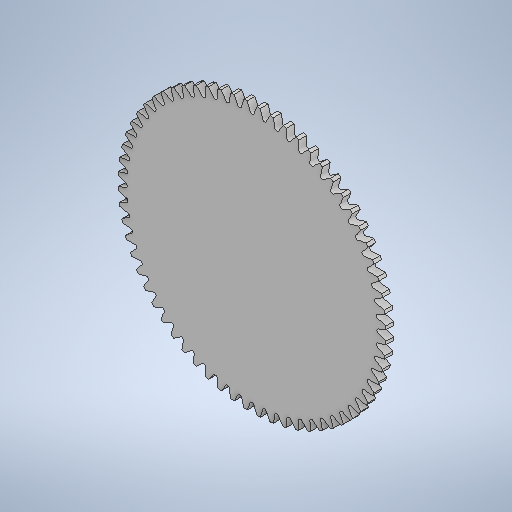
# Autodesk Inventor part: big gear
Saved by Autodesk Inventor 2025 (Build 290162010, 162A)
## iProperties
Created: 2025-08-27
Part Number: big gear
Material: Generic
Document SubType Name: Modeling
Designer: pokla
Density: 1 g/cm^3
Appearance: Default
Author: pokla
Autodesk Inventor part; units mm, degrees
ref_plane "YZ Plane" through (0, 0, 0) normal (1, 0, 0) x (0, 1, 0)
ref_plane "XZ Plane" through (0, 0, 0) normal (0, 1, 0) x (-1, 0, 0)
ref_plane "XY Plane" through (0, 0, 0) normal (0, 0, 1) x (1, 0, 0)
sketch "Sketch1" plane through (0, 0, 0) normal (0, 0, 1) x (1, 0, 0)
  spline S0 degree 3 poles (-15.3136, 412.2157) (-14.7005, 410.9627) (-13.4744, 408.4567) (-11.7613, 404.6382) (-10.1461, 400.7772) (-8.6557, 396.867) (-7.2691, 392.9165) (-6.406, 389.9001) (-5.7884, 387.899) (-5.3377, 386.951) (-4.8395, 386.2299) (-4.359, 385.7235) (-3.8332, 385.2647) (-3.236, 384.8928) (-2.5894, 384.6288) (-2.0848, 384.4891) (-1.5698, 384.3899) (-0.8714, 384.3654) (0, 384.3814) (0.8714, 384.3654) (1.5698, 384.3899) (2.0848, 384.4891) (2.5894, 384.6288) (3.236, 384.8928) (3.8332, 385.2647) (4.359, 385.7235) (4.8395, 386.2299) (5.3377, 386.951) (5.7884, 387.899) (6.406, 389.9001) (7.2691, 392.9165) (8.6557, 396.867) (10.1461, 400.7772) (11.7613, 404.6382) (13.4744, 408.4567) (14.7005, 410.9627) (15.3136, 412.2157) knots 0 0 0 0 0.418453 0.836906 1.255357 1.673806 2.09225 2.510695 2.615288 2.719831 2.824322 2.876636 2.92893 3.033403 3.085707 3.138007 3.190298 3.242598 3.347213 3.451829 3.504129 3.55642 3.60872 3.661023 3.765497 3.817791 3.870105 3.974596 4.079139 4.183732 4.602176 5.020621 5.43907 5.857521 6.275974 6.694427 6.694427 6.694427 6.694427
  circle A0 centre (0, 0) radius 384.375 construction
  circle A1 centre (0, 0) radius 375.877 construction
  circle A2 centre (0, 0) radius 400 construction
  circle A3 centre (0, 0) radius 412.5
  point P0 (-13.4954, 408.4468)
  point P1 (-11.7776, 404.6311)
  point P2 (-10.1669, 400.769)
  point P3 (-8.673, 396.8603)
  point P4 (-7.3084, 392.9046)
  point P5 (-6.0957, 388.8997)
  point P6 (-5.7647, 387.9075)
  point P7 (-5.3131, 386.9647)
  point P8 (-4.7127, 386.1094)
  point P9 (-4.3533, 385.7294)
  point P10 (-3.9585, 385.3864)
  point P11 (-3.0706, 384.8359)
  point P12 (-2.5862, 384.6385)
  point P13 (-2.083, 384.4958)
  point P14 (-1.5684, 384.4034)
  point P15 (-1.0462, 384.3746)
  point P16 (0, 384.375)
  point P17 (1.0462, 384.3746)
  point P18 (1.5684, 384.4034)
  point P19 (2.083, 384.4958)
  point P20 (2.5862, 384.6385)
  point P21 (3.0706, 384.8359)
  point P22 (3.9585, 385.3864)
  point P23 (4.3533, 385.7294)
  point P24 (4.7127, 386.1094)
  point P25 (5.3131, 386.9647)
  point P26 (5.7647, 387.9075)
  point P27 (6.0957, 388.8997)
  point P28 (7.3084, 392.9046)
  point P29 (8.673, 396.8603)
  point P30 (10.1669, 400.769)
  point P31 (11.7776, 404.6311)
  point P32 (13.4954, 408.4468)
  constraints: 4 centre point, 2 point on circle, 75 other
extrude "Extrusion1" add sketch "Sketch1" against normal blind 24
extrude "Extrusion2" cut sketch "Sketch1" against normal through all contours A3 S0 picked at (-1.5801, 403.5429)
pattern_circular "Circular Pattern1" count 64 over 360 about axis through (0, 0, -10) along (0, 0, 1) of "Extrusion2"
equation "\"Module\" = 12.5"
equation "\"PressureAngle\" = 20deg"
equation "\"UnitProfileClearance\" = 0.25"
equation "\"UnitRoundRadius\" = 0.35"
equation "\"HeadDiameter\" = 825"
equation "\"RootDiameter\" = 768.75"
equation "\"BaseDiameter\" = 751.7541"
equation "\"HelixAngle\" = 0"
equation "\"UnitCorrection\" = 0"
equation "\"UnitAddendumModification\" = 0"
equation "\"CircularPitch\" = 39.269908"
equation "\"UnitBacklashShift\" = 0"
equation "\"TotalToolShift\" = 0"
equation "\"IsInternal\" = 0"
body "Solid1"
